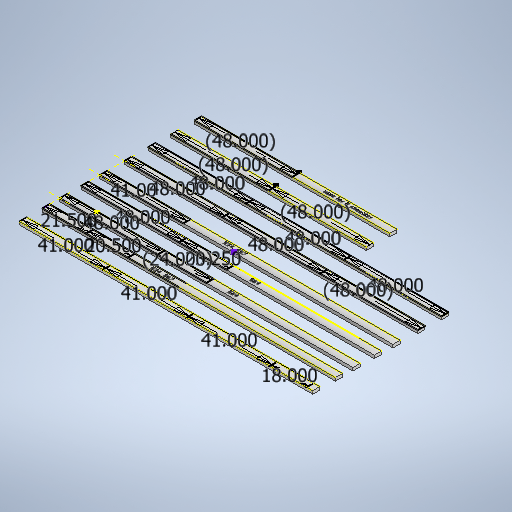
# Autodesk Inventor part: Lshoulder cuts
Saved by Autodesk Inventor 2026.1 (Build 301233000, 233)
## iProperties
Created: 2025-10-17
Part Number: Lshoulder cuts
Material: Generic
Document SubType Name: Modeling
Designer: jorda
Density: 1 g/cm^3
Appearance: Default
Author: jorda
Autodesk Inventor part; units mm, degrees
ref_plane "YZ Plane" through (0, 0, 0) normal (1, 0, 0) x (0, 1, 0)
ref_plane "XZ Plane" through (0, 0, 0) normal (0, 1, 0) x (-1, 0, 0)
ref_plane "XY Plane" through (0, 0, 0) normal (0, 0, 1) x (1, 0, 0)
sketch "Sketch1" plane through (0, 0, 0) normal (0, 1, 0) x (-1, 0, 0)
  line L0 (385.9062, 574.5992) -> (-3271.6938, 574.5992)
  line L1 (-3271.6938, 574.5992) -> (-3271.6938, 485.6992)
  line L2 (-3271.6938, 485.6992) -> (385.9062, 485.6992)
  line L3 (385.9062, 485.6992) -> (385.9062, 574.5992)
  line L4 (385.9062, 290.8577) -> (-3271.6938, 290.8577)
  line L5 (-3271.6938, 290.8577) -> (-3271.6938, 201.9577)
  line L6 (-3271.6938, 201.9577) -> (385.9062, 201.9577)
  line L7 (385.9062, 201.9577) -> (385.9062, 290.8577)
  line L8 (385.9062, 72.812) -> (-3271.6938, 72.812)
  line L9 (-3271.6938, 72.812) -> (-3271.6938, -16.088)
  line L10 (-3271.6938, -16.088) -> (385.9062, -16.088)
  line L11 (385.9062, -16.088) -> (385.9062, 72.812)
  line L12 (385.9062, -194.7435) -> (-3271.6938, -194.7435)
  line L13 (-3271.6938, -194.7435) -> (-3271.6938, -283.6435)
  line L14 (-3271.6938, -283.6435) -> (385.9062, -283.6435)
  line L15 (385.9062, -283.6435) -> (385.9062, -194.7435)
  line L16 (385.9062, -426.6687) -> (-3271.6938, -426.6687)
  line L17 (-3271.6938, -426.6687) -> (-3271.6938, -515.5687)
  line L18 (-3271.6938, -515.5687) -> (385.9062, -515.5687)
  line L19 (385.9062, -515.5687) -> (385.9062, -426.6687)
  line L20 (385.9062, -736.3666) -> (-3271.6938, -736.3666)
  line L21 (-3271.6938, -736.3666) -> (-3271.6938, -825.2666)
  line L22 (-3271.6938, -825.2666) -> (385.9062, -825.2666)
  line L23 (385.9062, -825.2666) -> (385.9062, -736.3666)
  line L24 (385.9062, -1031.6599) -> (-3271.6938, -1031.6599)
  line L25 (-3271.6938, -1031.6599) -> (-3271.6938, -1120.5599)
  line L26 (-3271.6938, -1120.5599) -> (385.9062, -1120.5599)
  line L27 (385.9062, -1120.5599) -> (385.9062, -1031.6599)
  line L28 (385.9062, -1312.5487) -> (-2052.4938, -1312.5487)
  line L29 (-2052.4938, -1312.5487) -> (-2052.4938, -1401.4487)
  line L30 (-2052.4938, -1401.4487) -> (385.9062, -1401.4487)
  line L31 (385.9062, -1401.4487) -> (385.9062, -1312.5487)
  line L32 (385.9062, -1607.8421) -> (-2052.4938, -1607.8421)
  line L33 (-2052.4938, -1607.8421) -> (-2052.4938, -1696.7421)
  line L34 (-2052.4938, -1696.7421) -> (385.9062, -1696.7421)
  line L35 (385.9062, -1696.7421) -> (385.9062, -1607.8421)
  point P0 (0, 0)
  constraints: 72 end point, 18 parallel, 9 horizontal, 9 perpendicular, 1 point on line
extrude "Extrusion1" add sketch "Sketch1" along normal blind 38.1
sketch "Sketch2" plane through (0, 38.1, 0) normal (0, 1, 0) x (1, 0, 0)
  line L0 (-385.9062, -574.5992) -> (3271.6938, -574.5992) projected
  line L1 (3271.6938, -485.6992) -> (-385.9062, -485.6992) projected
  line L2 (-385.9062, -574.5992) -> (655.4938, -574.5992)
  line L3 (655.4938, -574.5992) -> (655.4938, -485.6992)
  line L4 (655.4938, -485.6992) -> (-385.9062, -485.6992)
  line L5 (-385.9062, -485.6992) -> (-385.9062, -574.5992)
  line L6 (655.4938, -574.5992) -> (1696.8938, -574.5992)
  line L7 (1696.8938, -574.5992) -> (1696.8938, -485.6992)
  line L8 (1696.8938, -485.6992) -> (655.4938, -485.6992)
  line L9 (655.4938, -485.6992) -> (655.4938, -574.5992)
  line L10 (1696.8938, -574.5992) -> (2738.2938, -574.5992)
  line L11 (2738.2938, -574.5992) -> (2738.2938, -485.6992)
  line L12 (2738.2938, -485.6992) -> (1696.8938, -485.6992)
  line L13 (1696.8938, -485.6992) -> (1696.8938, -574.5992)
  line L14 (2738.2938, -574.5992) -> (3195.4938, -574.5992)
  line L15 (3195.4938, -574.5992) -> (3195.4938, -485.6992)
  line L16 (3195.4938, -485.6992) -> (2738.2938, -485.6992)
  line L17 (2738.2938, -485.6992) -> (2738.2938, -574.5992)
  point P0 (0, 0)
  dimension "d14" = 1041.4
  dimension "d15" = 1041.4
  dimension "d16" = 1041.4
  dimension "d17" = 457.2
  constraints: 32 end point, 8 parallel, 4 horizontal, 4 perpendicular, 4 point on line
  measures "d14" distance of L4.end L3.end
  measures "d15" distance of L8.end L7.end
  measures "d16" distance of L12.end L11.end
  measures "d17" distance of L16.end L15.end
sketch "Sketch3" plane through (0, 38.1, 0) normal (0, 1, 0) x (1, 0, 0)
  point P0 (0, 0)
sketch "Sketch4" plane through (0, 38.1, 0) normal (0, 1, 0) x (1, 0, 0)
  line L0 (-385.9062, 1312.5487) -> (2052.4938, 1312.5487) projected
  line L1 (-385.9062, 1312.5487) -> (833.2938, 1312.5487)
  line L2 (833.2938, 1312.5487) -> (744.3938, 1312.5487)
  line L3 (833.2938, 1312.5487) -> (833.2938, 1401.4487)
  line L4 (2052.4938, 1401.4487) -> (-385.9062, 1401.4487) projected
  line L5 (-385.9062, 1607.8421) -> (2052.4938, 1607.8421) projected
  line L6 (2052.4938, 1696.7421) -> (-385.9062, 1696.7421) projected
  line L7 (-385.9062, 1607.8421) -> (833.2938, 1607.8421)
  line L8 (833.2938, 1607.8421) -> (833.2938, 1696.7421)
  line L9 (833.2938, 1696.7421) -> (-385.9062, 1696.7421)
  line L10 (-385.9062, 1696.7421) -> (-385.9062, 1607.8421)
  line L11 (1180.5013, 1687.0985) -> (2076.0674, 1687.0985) construction
  line L12 (2076.0674, 1687.0985) -> (2076.0674, 1614.1334) construction
  line L13 (2076.0674, 1614.1334) -> (1180.5013, 1614.1334) construction
  line L14 (1180.5013, 1614.1334) -> (1180.5013, 1687.0985) construction
  point P0 (0, 0)
  dimension "d20" = 1219.2
  dimension "d21" = 1219.2
  dimension "d22" = 1219.2
  constraints: 14 end point, 6 midpoint, 2 parallel, 1 horizontal, 1 perpendicular, 1 point on line, 2 other
  measures "d20" distance of L4.end point (833.294, 1401.449)
  measures "d21" distance of L4.start point (833.294, 1401.449)
  measures "d22" distance of point (833.294, 1696.742) L6.end
sketch "Sketch5" plane through (0, 38.1, 0) normal (0, 1, 0) x (1, 0, 0)
  line L0 (-385.9062, -290.8577) -> (3271.6938, -290.8577) projected
  line L1 (3271.6938, -201.9577) -> (-385.9062, -201.9577) projected
  line L2 (-385.9062, -290.8577) -> (1315.8938, -290.8577)
  line L3 (1315.8938, -201.9577) -> (-385.9062, -201.9577)
  line L4 (-385.9062, -201.9577) -> (-385.9062, -290.8577)
  line L5 (-385.9062, -290.8577) -> (160.1938, -290.8577)
  line L6 (160.1938, -290.8577) -> (160.1938, -201.9577)
  line L7 (160.1938, -201.9577) -> (-385.9062, -201.9577)
  line L8 (-385.9062, -201.9577) -> (-385.9062, -290.8577)
  line L9 (160.1938, -290.8577) -> (680.8938, -290.8577)
  line L10 (680.8938, -290.8577) -> (680.8938, -201.9577)
  line L11 (680.8938, -201.9577) -> (160.1938, -201.9577)
  line L12 (160.1938, -201.9577) -> (160.1938, -290.8577)
  line L13 (932.1842, -223.6309) -> (1676.0985, -223.6309) construction
  line L14 (1676.0985, -223.6309) -> (1676.0985, -290.8577) construction
  line L15 (1676.0985, -290.8577) -> (932.1842, -290.8577) construction
  line L16 (932.1842, -290.8577) -> (932.1842, -223.6309) construction
  line L17 (3271.6938, 16.088) -> (-385.9062, 16.088) projected
  line L18 (-385.9062, -72.812) -> (833.2938, -72.812)
  line L19 (833.2938, -72.812) -> (833.2938, 16.088)
  line L20 (833.2938, 16.088) -> (-385.9062, 16.088)
  line L21 (-385.9062, 16.088) -> (-385.9062, -72.812)
  line L22 (833.2938, -72.812) -> (1442.8938, -72.812)
  line L23 (1442.8938, -72.812) -> (1442.8938, 16.088)
  line L24 (1442.8938, 16.088) -> (833.2938, 16.088)
  line L25 (833.2938, 16.088) -> (833.2938, -72.812)
  line L26 (1670.5598, 2.7748) -> (2044.3097, 2.7748) construction
  line L27 (2044.3097, 2.7748) -> (2044.3097, -71.9751) construction
  line L28 (2044.3097, -71.9751) -> (1670.5598, -71.9751) construction
  line L29 (1670.5598, -71.9751) -> (1670.5598, 2.7748) construction
  line L30 (1674.5456, 270.567) -> (2048.2955, 270.567) construction
  line L31 (2048.2955, 270.567) -> (2048.2955, 195.8171) construction
  line L32 (2048.2955, 195.8171) -> (1674.5456, 195.8171) construction
  line L33 (1674.5456, 195.8171) -> (1674.5456, 270.567) construction
  line L34 (-385.9062, 283.6435) -> (-385.9062, 194.7435) projected
  line L35 (3271.6938, 283.6435) -> (-385.9062, 283.6435) projected
  line L36 (-385.9062, 194.7435) -> (833.2938, 194.7435)
  line L37 (833.2938, 194.7435) -> (833.2938, 283.6435)
  line L38 (833.2938, 283.6435) -> (-385.9062, 283.6435)
  line L39 (-385.9062, 283.6435) -> (-385.9062, 194.7435)
  line L40 (3271.6938, 515.5687) -> (-385.9062, 515.5687) projected
  line L41 (-385.9062, 426.6687) -> (655.4938, 426.6687)
  line L42 (655.4938, 426.6687) -> (655.4938, 515.5687)
  line L43 (655.4938, 515.5687) -> (-385.9062, 515.5687)
  line L44 (-385.9062, 515.5687) -> (-385.9062, 426.6687)
  line L45 (1112.7606, 503.511) -> (1856.6748, 503.511) construction
  line L46 (1856.6748, 503.511) -> (1856.6748, 436.2841) construction
  line L47 (1856.6748, 436.2841) -> (1112.7606, 436.2841) construction
  line L48 (1112.7606, 436.2841) -> (1112.7606, 503.511) construction
  line L49 (3271.6938, 825.2666) -> (-385.9062, 825.2666) projected
  line L50 (-385.9062, 736.3666) -> (833.2938, 736.3666)
  line L51 (833.2938, 736.3666) -> (833.2938, 825.2666)
  line L52 (833.2938, 825.2666) -> (-385.9062, 825.2666)
  line L53 (-385.9062, 825.2666) -> (-385.9062, 736.3666)
  line L54 (833.2938, 736.3666) -> (2052.4938, 736.3666)
  line L55 (2052.4938, 736.3666) -> (2052.4938, 825.2666)
  line L56 (2052.4938, 825.2666) -> (833.2938, 825.2666)
  line L57 (833.2938, 825.2666) -> (833.2938, 736.3666)
  line L58 (2052.4938, 736.3666) -> (3271.6938, 736.3666)
  line L59 (3271.6938, 736.3666) -> (3271.6938, 825.2666)
  line L60 (3271.6938, 825.2666) -> (2052.4938, 825.2666)
  line L61 (2052.4938, 825.2666) -> (2052.4938, 736.3666)
  line L62 (3271.6938, 1031.6599) -> (3271.6938, 1120.5599) projected
  line L63 (-385.9062, 1031.6599) -> (3271.6938, 1031.6599) projected
  line L64 (3271.6938, 1120.5599) -> (2052.4938, 1120.5599)
  line L65 (2052.4938, 1120.5599) -> (2052.4938, 1031.6599)
  line L66 (2052.4938, 1031.6599) -> (3271.6938, 1031.6599)
  line L67 (3271.6938, 1031.6599) -> (3271.6938, 1120.5599)
  line L68 (2052.4938, 1120.5599) -> (833.2938, 1120.5599)
  line L69 (833.2938, 1120.5599) -> (833.2938, 1031.6599)
  line L70 (833.2938, 1031.6599) -> (2052.4938, 1031.6599)
  line L71 (2052.4938, 1031.6599) -> (2052.4938, 1120.5599)
  line L72 (833.2938, 1031.6599) -> (-385.9062, 1031.6599)
  line L73 (-385.9062, 1031.6599) -> (-385.9062, 1120.5599)
  line L74 (-385.9062, 1120.5599) -> (833.2938, 1120.5599)
  line L75 (833.2938, 1120.5599) -> (833.2938, 1031.6599)
  line L76 (833.2938, 194.7435) -> (1423.8438, 194.7435)
  line L77 (1423.8438, 194.7435) -> (1423.8438, 283.6435)
  line L78 (1423.8438, 283.6435) -> (833.2938, 283.6435)
  line L79 (833.2938, 283.6435) -> (833.2938, 194.7435)
  point P0 (1278.9754, 436.2841)
  dimension "d24" = 546.1
  dimension "d25" = 520.7
  dimension "d27" = 1219.2
  dimension "d28" = 609.6
  dimension "d29" = 1219.2
  dimension "d30" = 1041.4
  dimension "d31" = 1219.2
  dimension "d32" = 1219.2
  dimension "d33" = 1219.2
  dimension "d34" = 1219.2
  dimension "d35" = 1219.2
  dimension "d36" = 1219.2
  dimension "d37" = 590.55
  constraints: 110 end point, 27 parallel, 14 horizontal, 14 point on line, 13 perpendicular, 1 midpoint, 8 other
  measures "d24" distance of L7.end L6.end
  measures "d25" distance of L11.end L10.end
  measures "d27" distance of L20.end L19.end
  measures "d28" distance of L24.end L23.end
  measures "d29" distance of L37.end L34.start
  measures "d30" distance of L43.end L42.end
  measures "d31" distance of L52.end L51.end
  measures "d32" distance of L56.end L55.end
  measures "d33" distance of L49.start L55.end
  measures "d34" distance of L68.end L73.end
  measures "d35" distance of L64.end L68.end
  measures "d36" distance of L62.end L64.end
  measures "d37" distance of L78.end L77.end
body "Solid1"
